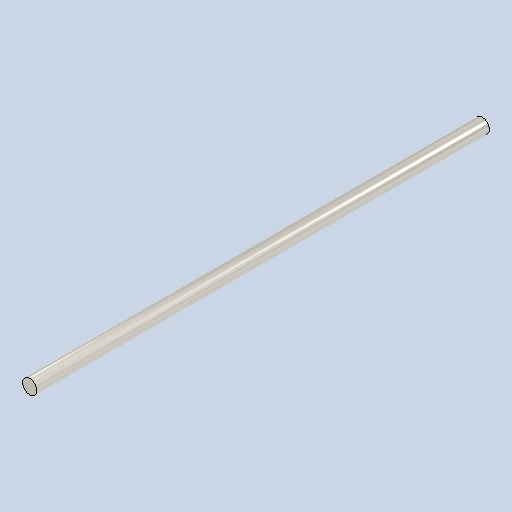
# Autodesk Inventor part: w-wire-10
Saved by Autodesk Inventor 2026 (Build 300175050, 175E)
## iProperties
Created: 2025-08-20
Part Number: w-wire-10
Material: Titanium
Document SubType Name: Modeling
Designer: kuzmin
Density: 4.51 g/cm^3
Appearance: Titanium
Author: kuzmin
Autodesk Inventor part; units mm, degrees
ref_plane "YZ Plane" through (0, 0, 0) normal (1, 0, 0) x (0, 1, 0)
ref_plane "XZ Plane" through (0, 0, 0) normal (0, 1, 0) x (-1, 0, 0)
ref_plane "XY Plane" through (0, 0, 0) normal (0, 0, 1) x (1, 0, 0)
sketch "Sketch1" plane through (0, 0, 0) normal (0, 0, 1) x (1, 0, 0)
  circle A0 centre (0, 0) radius 0.25
  dimension "d0" = 0.5
  constraints: 1 centre point, 1 coincident
  measures "d0" diameter of A0
extrude "Extrusion1" add sketch "Sketch1" along normal blind 16
body "Solid1"
